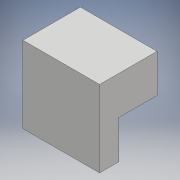
# Autodesk Inventor part: CarroXY - FimCurso
Saved by Autodesk Inventor 2017 (Build 210142000, 142)
## iProperties
Created: 2020-08-19
Part Number: CarroXY - FimCurso
Material: Generic
Document SubType Name: Modeling
Designer: ale
Density: 1 g/cm^3
Appearance: Default
Author: ale
Autodesk Inventor part; units mm, degrees
ref_plane "YZ Plane" through (0, 0, 0) normal (1, 0, 0) x (0, 1, 0)
ref_plane "XZ Plane" through (0, 0, 0) normal (0, 1, 0) x (-1, 0, 0)
ref_plane "XY Plane" through (0, 0, 0) normal (0, 0, 1) x (1, 0, 0)
sketch "Sketch1" plane through (0, 0, 0) normal (0, 0, 1) x (1, 0, 0)
  line L0 (-6, -3) -> (6, -3)
  line L1 (6, -3) -> (6, 3)
  line L2 (6, 3) -> (-6, 3)
  line L3 (-6, 3) -> (-6, -3)
  line L4 (-6, -3) -> (6, 3) construction
  line L5 (6, -3) -> (-6, 3) construction
  point P0 (0, 0)
  dimension "d0" = 12
  dimension "d1" = 6
  constraints: 12 end point, 2 midpoint, 2 parallel, 1 horizontal, 1 perpendicular
  measures "d0" distance of L2.end L1.end
  measures "d1" distance of L1.end L0.end
extrude "Extrusion1" add sketch "Sketch1" along normal blind 6
sketch "Sketch2" plane through (-6, -3, 0) normal (0, -1, 0) x (1, 0, 0)
  line L0 (0, 6) -> (12, 6) projected
  line L1 (12, 6) -> (0, 6)
  line L2 (0, 6) -> (0, -6)
  line L3 (0, -6) -> (12, -6)
  line L4 (12, -6) -> (12, 6)
  point P0 (6, 0)
  dimension "d4" = 12
  dimension "d5" = 12
  constraints: 8 end point, 2 parallel, 1 horizontal, 1 perpendicular
  measures "d4" distance of L3.end L2.end
  measures "d5" distance of L2.end L1.end
extrude "Extrusion2" add sketch "Sketch2" along normal blind 3
body "Solid1"
